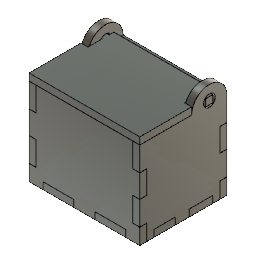
Music Box v1 (Autodesk Fusion 360 design; units mm, degrees)
Autodesk Fusion 360 part; units mm, degrees
sketch "Sketch1" plane through (0, 0, 0) normal (0, 0, 1) x (1, 0, 0)
  line L0 (0, 0) -> (47, 0)
  line L1 (47, 0) -> (47, 37)
  line L2 (47, 37) -> (0, 37)
  line L3 (0, 37) -> (0, 0)
  dimension "d1" = 47
  dimension "d2" = 37
  constraint horizontal L0
  constraint vertical L1
  constraint horizontal L2
  constraint vertical L3
  constraint coincident L0.start L3.end
  measures "d1" distance of L0.start L0.end
  measures "d2" distance of L0.start L2.end
sketch "Sketch2" plane through (0, 0, 0) normal (0, 0, 1) x (1, 0, 0)
  line L0 (0, 0) -> (3, 0)
  line L1 (3, 0) -> (3, 3)
  line L2 (3, 3) -> (0, 3)
  line L3 (0, 3) -> (0, 0)
  line L4 (25, 0) -> (25, 3)
  line L5 (22, 0) -> (25, 0)
  line L6 (25, 3) -> (22, 3)
  line L7 (22, 3) -> (22, 0)
  line L8 (47, 0) -> (47, 3)
  line L9 (44, 0) -> (47, 0)
  line L10 (47, 3) -> (44, 3)
  line L11 (44, 3) -> (44, 0)
  line L12 (25, 0) -> (28, 0)
  line L13 (28, 0) -> (28, 3)
  line L14 (25, 3) -> (25, 0)
  line L15 (28, 3) -> (25, 3)
  line L16 (22, 3) -> (19, 3)
  line L17 (22, 3) -> (22, 0)
  line L18 (19, 0) -> (22, 0)
  line L19 (19, 3) -> (19, 0)
  line L20 (6, 3) -> (3, 3)
  line L21 (6, 0) -> (6, 3)
  line L22 (3, 0) -> (6, 0)
  line L23 (3, 3) -> (3, 0)
  line L24 (41, 3) -> (41, 0)
  line L25 (44, 3) -> (41, 3)
  line L26 (41, 0) -> (44, 0)
  line L27 (44, 0) -> (44, 3)
  line L28 (19, 37) -> (19, 34)
  line L29 (28, 34) -> (28, 37)
  line L30 (25, 34) -> (28, 34)
  line L31 (22, 34) -> (25, 34)
  line L32 (28, 37) -> (25, 37)
  line L33 (25, 37) -> (22, 37)
  line L34 (22, 37) -> (19, 37)
  line L35 (6, 37) -> (3, 37)
  line L36 (6, 34) -> (6, 37)
  line L37 (3, 34) -> (6, 34)
  line L38 (0, 34) -> (3, 34)
  line L39 (0, 37) -> (0, 34)
  line L40 (3, 37) -> (0, 37)
  line L41 (41, 37) -> (41, 34)
  line L42 (44, 37) -> (41, 37)
  line L43 (47, 37) -> (44, 37)
  line L44 (41, 34) -> (44, 34)
  line L45 (44, 34) -> (47, 34)
  line L46 (47, 34) -> (47, 37)
  line L47 (19, 34) -> (22, 34)
  line L48 (47, 0) -> (47, 3)
  line L49 (47, 3) -> (44, 3)
  line L50 (44, 3) -> (44, 0)
  line L51 (44, 0) -> (47, 0)
  line L52 (3, 31) -> (3, 34)
  line L53 (3, 34) -> (0, 34)
  line L54 (0, 34) -> (0, 31)
  line L55 (0, 31) -> (3, 31)
  line L56 (47, 31) -> (47, 34)
  line L57 (47, 34) -> (44, 34)
  line L58 (44, 34) -> (44, 31)
  line L59 (44, 31) -> (47, 31)
  line L60 (3, 3) -> (3, 6)
  line L61 (0, 3) -> (3, 3)
  line L62 (0, 6) -> (0, 3)
  line L63 (3, 6) -> (0, 6)
  line L64 (44, 6) -> (44, 3)
  line L65 (44, 3) -> (47, 3)
  line L66 (47, 6) -> (44, 6)
  line L67 (47, 3) -> (47, 6)
  line L68 (44, 15) -> (47, 15)
  line L69 (47, 15) -> (47, 18)
  line L70 (47, 18) -> (47, 21)
  line L71 (47, 21) -> (44, 21)
  line L72 (44, 21) -> (44, 18)
  line L73 (44, 15) -> (44, 18)
  line L74 (3, 18) -> (3, 21)
  line L75 (3, 21) -> (0, 21)
  line L76 (0, 21) -> (0, 18)
  line L77 (0, 18) -> (0, 15)
  line L78 (0, 15) -> (3, 15)
  line L79 (3, 18) -> (3, 15)
  point P0 (0, 6)
  dimension "d9" = 3
  dimension "d10" = 3
  dimension "d13" = 44
  dimension "d14" = 0
  dimension "d17" = 3
  dimension "d18" = 0
  dimension "d21" = -3
  dimension "d22" = 0
  dimension "d25" = 3
  dimension "d26" = 0
  dimension "d29" = -3
  dimension "d30" = 0
  dimension "d33" = 0
  dimension "d34" = 34
  dimension "d37" = 44
  dimension "d38" = 31
  dimension "d41" = 0
  dimension "d42" = -28
  dimension "d45" = 0
  dimension "d46" = 15
  constraint horizontal L0
  constraint vertical L1
  constraint horizontal L2
  constraint vertical L3
  constraint coincident L0.start L3.end
  measures "d9" distance of L0.start L0.end
  measures "d10" distance of L0.start L2.end
extrude "Extrude1" add sketch "Sketch1" along normal blind 3 makes body 1
extrude "Extrude2" cut sketch "Sketch2" along normal blind 3 bodies 1
sketch "Sketch3" plane through (0, 0, 0) normal (0, 0, 1) x (1, 0, 0)
  line L0 (0, 0) -> (47, 0)
  line L1 (47, 0) -> (47, 3)
  line L2 (47, 3) -> (0, 3)
  line L3 (0, 3) -> (0, 0)
  dimension "d51" = 47
  dimension "d52" = 3
  constraint horizontal L0
  constraint vertical L1
  constraint horizontal L2
  constraint vertical L3
  constraint coincident L0.start L3.end
  measures "d51" distance of L0.start L0.end
  measures "d52" distance of L0.start L2.end
extrude "Extrude1'" add sketch "Sketch3" along normal blind 37 separate body makes body 2 in component "Component"
sketch "Sketch4" plane through (0, 0, 0) normal (0, -1, 0) x (1, 0, 0)
  line L0 (0, 0) -> (47, 0)
  line L1 (47, 0) -> (47, 37)
  line L2 (47, 37) -> (0, 37)
  line L3 (0, 37) -> (0, 0)
  line L4 (0, 37) -> (3, 37)
  line L5 (3, 37) -> (3, 26.7867)
  line L6 (3, 26.7867) -> (0, 26.7867)
  line L7 (0, 26.7867) -> (0, 37)
  line L8 (44, 37) -> (47, 37)
  line L9 (47, 37) -> (47, 26.7867)
  line L10 (44, 26.7867) -> (44, 37)
  line L11 (47, 26.7867) -> (44, 26.7867)
  line L12 (0, 17) -> (3, 17)
  line L13 (3, 17) -> (3, 6.7867)
  line L14 (0, 6.7867) -> (0, 17)
  line L15 (3, 6.7867) -> (0, 6.7867)
  line L16 (44, 17) -> (47, 17)
  line L17 (47, 17) -> (47, 6.7867)
  line L18 (44, 6.7867) -> (44, 17)
  line L19 (47, 6.7867) -> (44, 6.7867)
  line L20 (19, 0) -> (6, 0)
  line L21 (6, 0) -> (6, 3)
  line L22 (6, 3) -> (19, 3)
  line L23 (19, 3) -> (19, 0)
  line L24 (41, 3) -> (41, 0)
  line L25 (41, 0) -> (28, 0)
  line L26 (28, 3) -> (41, 3)
  line L27 (28, 0) -> (28, 3)
  dimension "d55" = 3
  dimension "d56" = 10.2133
  dimension "d59" = 44
  dimension "d60" = -20
  dimension "d61" = 13
  dimension "d62" = 3
  dimension "d65" = 22
  dimension "d66" = 0
  constraint horizontal L4
  constraint vertical L5
  constraint horizontal L6
  constraint vertical L7
  constraint coincident L2.end L3.start
  constraint horizontal L20
  constraint vertical L21
  constraint horizontal L22
  constraint vertical L23
  constraint coincident L0 L20.start
  measures "d55" distance of L2.end L4.end
  measures "d56" distance of L2.end L6.end
  measures "d61" distance of L20.start L20.end
  measures "d62" distance of L20.start L22.end
extrude "Extrude2'" cut sketch "Sketch4" against normal blind 3 contours L0 L20 L21 L22 L23 | L3 L12 L13 L14 L15 | L0 L24 L25 L26 L27 | L2 L3 L4 L5 L6 L7 | L1 L16 L17 L18 L19 | L1 L2 L8 L9 L10 L11 bodies 2 in component "Component"
sketch "Sketch5" plane through (0, 0, 0) normal (-1, 0, 0) x (0, -1, 0)
  line L0 (0, 26.7867) -> (-3, 26.7867)
  line L1 (-3, 26.7867) -> (-3, 17)
  line L2 (-3, 17) -> (0, 17)
  line L3 (0, 17) -> (0, 26.7867)
  line L4 (0, 0) -> (-37, 0)
  line L5 (-37, 0) -> (-37, 37)
  line L6 (-37, 37) -> (0, 37)
  line L7 (0, 37) -> (0, 0)
  line L8 (0, 6.816) -> (-3, 6.816)
  line L9 (-3, 6.816) -> (-3, 0)
  line L10 (-3, 0) -> (0, 0)
  line L11 (0, 0) -> (0, 6.816)
  dimension "d69" = 37
  dimension "d70" = 37
  constraint horizontal L4
  constraint vertical L5
  constraint horizontal L6
  constraint vertical L7
  constraint coincident L4.start L7.end
  constraint horizontal L8
  constraint vertical L9
  constraint horizontal L10
  constraint vertical L11
  constraint coincident L4 L9.end
  constraint coincident L7 L8.start
  measures "d69" distance of L4.start L4.end
  measures "d70" distance of L4.start L6.end
sketch "Sketch6" plane through (0, 0, 0) normal (-1, 0, 0) x (0, -1, 0)
  line L0 (-3, 6.816) -> (0, 6.816)
  line L1 (0, 6.816) -> (0, 17)
  line L2 (0, 17) -> (-3, 17)
  line L3 (-3, 17) -> (-3, 26.7867)
  line L4 (-3, 26.7867) -> (0, 26.7867)
  line L5 (0, 26.7867) -> (0, 37)
  line L6 (0, 37) -> (-37, 37)
  line L7 (-37, 37) -> (-37, 0)
  line L8 (-37, 0) -> (-3, 0)
  line L9 (-3, 0) -> (-3, 6.816)
  line L10 (-37, 26.7867) -> (-34, 26.7867)
  line L11 (-37, 17) -> (-37, 26.7867)
  line L12 (-34, 17) -> (-37, 17)
  line L13 (-37, 6.816) -> (-34, 6.816)
  line L14 (-37, 0) -> (-37, 6.816)
  spline S0 degree 5 poles (-34, 26.7867) (-34, 26.3953) (-34, 25.6123) (-34, 24.4379) (-34, 22.872) (-34, 20.9147) (-34, 19.3488) (-34, 18.1744) (-34, 17.3915) (-34, 17) knots 0 0 0 0 0 0 0.2 0.4 0.6 0.8 1 1 1 1 1 1
  spline S1 degree 5 poles (-34, 6.816) (-34, 6.5433) (-34, 5.9981) (-34, 5.1801) (-34, 4.0896) (-34, 2.7264) (-34, 1.6358) (-34, 0.8179) (-34, 0.2726) (-34, 0) knots 0 0 0 0 0 0 0.2 0.4 0.6 0.8 1 1 1 1 1 1
  spline S2 degree 5 poles (-37, 0) (-36.88, 0) (-36.64, 0) (-36.28, 0) (-35.8, 0) (-35.2, 0) (-34.72, 0) (-34.36, 0) (-34.12, 0) (-34, 0) knots 0 0 0 0 0 0 0.2 0.4 0.6 0.8 1 1 1 1 1 1
  line L15 (-31, 3) -> (-26, 3)
  line L16 (-26, 3) -> (-26, 0)
  line L17 (-26, 0) -> (-31, 0)
  line L18 (-31, 0) -> (-31, 3)
  line L19 (-26, 3) -> (-21, 3)
  line L20 (-26, 0) -> (-26, 3)
  line L21 (-21, 3) -> (-21, 0)
  line L22 (-21, 0) -> (-26, 0)
  line L23 (-15, 0) -> (-12, 0)
  line L24 (-12, 0) -> (-12, 3)
  line L25 (-12, 3) -> (-15, 3)
  line L26 (-15, 3) -> (-15, 0)
  line L27 (-9, 3) -> (-12, 3)
  line L28 (-12, 3) -> (-12, 0)
  line L29 (-12, 0) -> (-9, 0)
  line L30 (-9, 0) -> (-9, 3)
  line L31 (-6, 3) -> (-9, 3)
  line L32 (-9, 3) -> (-9, 0)
  line L33 (-9, 0) -> (-6, 0)
  line L34 (-6, 0) -> (-6, 3)
  dimension "d75" = -34
  dimension "d76" = 0
  dimension "d77" = 5
  dimension "d78" = 3
  dimension "d81" = 5
  dimension "d82" = 0
  dimension "d83" = 3
  dimension "d84" = 3
  dimension "d87" = 6
  dimension "d88" = 0
  constraint coincident L8 S1.end
  constraint coincident L7.end L8.start
  constraint horizontal L15
  constraint vertical L16
  constraint horizontal L17
  constraint vertical L18
  constraint horizontal L23
  constraint vertical L24
  constraint horizontal L25
  constraint vertical L26
  measures "d77" distance of L15.start L15.end
  measures "d78" distance of L15.start L17.end
  measures "d83" distance of L23.start L23.end
  measures "d84" distance of L23.start L25.end
extrude "Extrude1''" add sketch "Sketch6" against normal blind 3 separate body contours L0 L1 L2 L3 L4 L5 L6 L7 L8 L9 L10 L12 L13 S0 S1 L15 L18 L19 L21 L25 L26 L27 L31 L34 makes body 3 in component "Component'"
extrude "Extrude1'''" add 1 faces at (22, 0, 18.8578) along direction (0, -1, 0) blind -37 and the other way blind 34 separate body on bodies 2 makes body 4 in component "Component''"
extrude "Extrude1''''" add 1 faces at (3, 19.3333, 12.3333) along direction (1, 0, 0) blind 41 and the other way blind -44 separate body on bodies 3 makes body 5 in component "Component'''"
extrude "Extrude3" cut 1 faces at (16.6667, 2, 37) along direction (0, 0, -1) blind 3 on bodies 2 bodies 2 in component "Component"
sketch "Sketch7" plane through (47, 0, 0) normal (1, 0, 0) x (0, 1, 0)
  line L0 (3, 6.816) -> (3, 0)
  line L1 (3, 0) -> (6, 0)
  line L2 (6, 0) -> (6, 3)
  line L3 (6, 3) -> (15, 3)
  line L4 (15, 3) -> (15, 0)
  line L5 (15, 0) -> (21, 0)
  line L6 (21, 0) -> (21, 3)
  line L7 (21, 3) -> (31, 3)
  line L8 (31, 3) -> (31, 0)
  line L9 (31, 0) -> (34, 0)
  line L10 (34, 0) -> (34, 6.816)
  line L11 (34, 6.816) -> (37, 6.816)
  line L12 (37, 6.816) -> (37, 17)
  line L13 (37, 17) -> (34, 17)
  line L14 (34, 17) -> (34, 26.7867)
  line L15 (34, 26.7867) -> (37, 26.7867)
  line L16 (37, 26.7867) -> (37, 37)
  line L17 (37, 37) -> (0, 37)
  line L18 (0, 37) -> (0, 26.7867)
  line L19 (0, 26.7867) -> (3, 26.7867)
  line L20 (3, 26.7867) -> (3, 17)
  line L21 (3, 17) -> (0, 17)
  line L22 (0, 17) -> (0, 6.816)
  line L23 (0, 6.816) -> (3, 6.816)
  circle A0 centre (29.5075, 37) radius 7.5
  dimension "d101" = 15
  constraint coincident L17 A0.centre
  measures "d101" diameter of A0
extrude "Extrude2''" add sketch "Sketch7" against normal blind 3 contours L16 L17 A0 picked at (27.0329, 37.3726) bodies 5 in component "Component'''"
sketch "Sketch8" plane through (0, 0, 0) normal (-1, 0, 0) x (0, -1, 0)
  line L0 (-3, 0) -> (-3, 6.816)
  line L1 (-3, 6.816) -> (0, 6.816)
  line L2 (0, 6.816) -> (0, 17)
  line L3 (0, 17) -> (-3, 17)
  line L4 (-3, 17) -> (-3, 26.7867)
  line L5 (-3, 26.7867) -> (0, 26.7867)
  line L6 (0, 26.7867) -> (0, 37)
  line L7 (0, 37) -> (-37, 37)
  line L8 (-37, 37) -> (-37, 26.7867)
  line L9 (-37, 26.7867) -> (-34, 26.7867)
  line L10 (-34, 26.7867) -> (-34, 17)
  line L11 (-34, 17) -> (-37, 17)
  line L12 (-37, 17) -> (-37, 6.816)
  line L13 (-37, 6.816) -> (-34, 6.816)
  line L14 (-34, 6.816) -> (-34, 0)
  line L15 (-34, 0) -> (-31, 0)
  line L16 (-31, 0) -> (-31, 3)
  line L17 (-31, 3) -> (-21, 3)
  line L18 (-21, 3) -> (-21, 0)
  line L19 (-21, 0) -> (-15, 0)
  line L20 (-15, 0) -> (-15, 3)
  line L21 (-15, 3) -> (-6, 3)
  line L22 (-6, 3) -> (-6, 0)
  line L23 (-6, 0) -> (-3, 0)
  circle A0 centre (-29.4944, 37) radius 7.5
  dimension "d104" = 15
  constraint coincident L7 A0.centre
  measures "d104" diameter of A0
extrude "Extrude2'''" add sketch "Sketch8" against normal blind 3 contours L7 A0 picked at (-30.0507, 39.4373) bodies 3 in component "Component'"
extrude "Extrude4" add 1 faces at (16.6667, 2, 34) along direction (0, 0, 1) blind 3 on bodies 2 bodies 2 in component "Component"
sketch "Sketch9" plane through (0, 0, 3) normal (0, 0, 1) x (-1, 0, 0)
  line L0 (-41, 0) -> (-41, -3)
  line L1 (-41, -3) -> (-44, -3)
  line L2 (-44, -3) -> (-44, -6)
  line L3 (-44, -6) -> (-47, -6)
  line L4 (-47, -6) -> (-47, -15)
  line L5 (-47, -15) -> (-44, -15)
  line L6 (-44, -15) -> (-44, -21)
  line L7 (-44, -21) -> (-47, -21)
  line L8 (-47, -21) -> (-47, -31)
  line L9 (-47, -31) -> (-44, -31)
  line L10 (-44, -31) -> (-44, -34)
  line L11 (-44, -34) -> (-41, -34)
  line L12 (-41, -34) -> (-41, -37)
  line L13 (-41, -37) -> (-28, -37)
  line L14 (-28, -37) -> (-28, -34)
  line L15 (-28, -34) -> (-19, -34)
  line L16 (-19, -34) -> (-19, -37)
  line L17 (-19, -37) -> (-6, -37)
  line L18 (-6, -37) -> (-6, -34)
  line L19 (-6, -34) -> (-3, -34)
  line L20 (-3, -34) -> (-3, -31)
  line L21 (-3, -31) -> (0, -31)
  line L22 (0, -31) -> (0, -21)
  line L23 (0, -21) -> (-3, -21)
  line L24 (-3, -21) -> (-3, -15)
  line L25 (-3, -15) -> (0, -15)
  line L26 (0, -15) -> (0, -6)
  line L27 (0, -6) -> (-3, -6)
  line L28 (-3, -6) -> (-3, -3)
  line L29 (-3, -3) -> (-6, -3)
  line L30 (-6, -3) -> (-6, 0)
  line L31 (-6, 0) -> (-19, 0)
  line L32 (-19, 0) -> (-19, -3)
  line L33 (-19, -3) -> (-28, -3)
  line L34 (-28, -3) -> (-28, 0)
  line L35 (-28, 0) -> (-41, 0)
  line L36 (0, 0) -> (-47, 0)
  line L37 (-47, 0) -> (-47, -37)
  line L38 (-47, -37) -> (0, -37)
  line L39 (0, -37) -> (0, 0)
  dimension "d109" = 47
  dimension "d110" = 37
  constraint horizontal L36
  constraint vertical L37
  constraint horizontal L38
  constraint vertical L39
  constraint coincident L36.start L39.end
  measures "d109" distance of L36.start L36.end
  measures "d110" distance of L36.start L38.end
extrude "Extrude1'''''" add sketch "Sketch9" along normal blind 37 and the other way blind -34 separate body makes body 6 in component "Component''''"
sketch "Sketch10" plane through (0, 0, 40) normal (0, 0, 1) x (-1, 0, 0)
  line L0 (0, -37) -> (0, 0)
  line L1 (0, 0) -> (-47, 0)
  line L2 (-47, 0) -> (-47, -37)
  line L3 (-47, -37) -> (0, -37)
  line L4 (0, -37) -> (-3, -37)
  line L5 (-3, -37) -> (-3, -22)
  line L6 (-3, -22) -> (0, -22)
  line L7 (0, -22) -> (0, -37)
  line L8 (-44, -37) -> (-47, -37)
  line L9 (-47, -37) -> (-47, -22)
  line L10 (-44, -22) -> (-44, -37)
  line L11 (-47, -22) -> (-44, -22)
  dimension "d117" = -44
  dimension "d118" = 0
  constraint horizontal L4
  constraint vertical L5
  constraint horizontal L6
  constraint vertical L7
  constraint coincident L0.start L3.end
extrude "Extrude2''''" cut sketch "Sketch10" against normal blind 3 contours L0 L3 L4 L5 L6 L7 | L2 L3 L8 L9 L10 L11 bodies 6 in component "Component''''"
sketch "Sketch11" plane through (0, 0, 40) normal (0, 0, 1) x (-1, 0, 0)
  line L0 (-3, -22) -> (0, -22)
  line L1 (0, -22) -> (0, 0)
  line L2 (0, 0) -> (-47, 0)
  line L3 (-47, 0) -> (-47, -22)
  line L4 (-47, -22) -> (-44, -22)
  line L5 (-44, -22) -> (-44, -37)
  line L6 (-44, -37) -> (-3, -37)
  line L7 (-3, -37) -> (-3, -22)
  line L8 (-3, -37) -> (-44, -37)
  line L9 (-44, -37) -> (-44, -34)
  line L10 (-44, -34) -> (-3, -34)
  line L11 (-3, -34) -> (-3, -37)
  dimension "d121" = 3
  constraint horizontal L8
  constraint vertical L9
  constraint horizontal L10
  constraint vertical L11
  constraint coincident L6.end L7.start
  measures "d121" distance of L6.end L10.end
extrude "Extrude3'" cut sketch "Sketch11" against normal blind 3 contours L5 L6 L7 L8 L9 L10 L11 bodies 6 in component "Component''''"
sketch "Sketch12" plane through (0, 0, 40) normal (0, 0, 1) x (-1, 0, 0)
  line L0 (-44, -34) -> (-3, -34)
  line L1 (-3, -34) -> (-3, -22)
  line L2 (-3, -22) -> (0, -22)
  line L3 (0, -22) -> (0, 0)
  line L4 (0, 0) -> (-47, 0)
  line L5 (-47, 0) -> (-47, -22)
  line L6 (-47, -22) -> (-44, -22)
  line L7 (-44, -22) -> (-44, -34)
hole "Hole1" at (47, 29.5396, 38.575) direction (-1, 0, 0) diameter 5 depth 49 tip angle 118 bodies 3 in component "Component'"
hole "Hole1'" at (47, 29.5396, 38.575) direction (-1, 0, 0) diameter 5 depth 49 tip angle 118 bodies 5 in component "Component'''"
sketch "Sketch13" plane through (0, 0, 40) normal (0, 0, 1) x (1, 0, 0)
  line L0 (3, 31) -> (0, 31)
  line L1 (0, 31) -> (0, 28)
  line L2 (0, 28) -> (3, 28)
  line L3 (3, 28) -> (3, 31)
  constraint horizontal L0
  constraint vertical L1
  constraint horizontal L2
  constraint vertical L3
extrude "Extrude4'" add sketch "Sketch13" against normal blind 3 bodies 6 in component "Component''''"
sketch "Sketch14" plane through (0, 0, 3) normal (0, 0, 1) x (-1, 0, 0)
  line L0 (-41, 0) -> (-41, -3)
  line L1 (-41, -3) -> (-44, -3)
  line L2 (-44, -3) -> (-44, -6)
  line L3 (-44, -6) -> (-47, -6)
  line L4 (-47, -6) -> (-47, -15)
  line L5 (-47, -15) -> (-44, -15)
  line L6 (-44, -15) -> (-44, -21)
  line L7 (-44, -21) -> (-47, -21)
  line L8 (-47, -21) -> (-47, -31)
  line L9 (-47, -31) -> (-44, -31)
  line L10 (-44, -31) -> (-44, -34)
  line L11 (-44, -34) -> (-41, -34)
  line L12 (-41, -34) -> (-41, -37)
  line L13 (-41, -37) -> (-28, -37)
  line L14 (-28, -37) -> (-28, -34)
  line L15 (-28, -34) -> (-19, -34)
  line L16 (-19, -34) -> (-19, -37)
  line L17 (-19, -37) -> (-6, -37)
  line L18 (-6, -37) -> (-6, -34)
  line L19 (-6, -34) -> (-3, -34)
  line L20 (-3, -34) -> (-3, -31)
  line L21 (-3, -31) -> (0, -31)
  line L22 (0, -31) -> (0, -21)
  line L23 (0, -21) -> (-3, -21)
  line L24 (-3, -21) -> (-3, -15)
  line L25 (-3, -15) -> (0, -15)
  line L26 (0, -15) -> (0, -6)
  line L27 (0, -6) -> (-3, -6)
  line L28 (-3, -6) -> (-3, -3)
  line L29 (-3, -3) -> (-6, -3)
  line L30 (-6, -3) -> (-6, 0)
  line L31 (-6, 0) -> (-19, 0)
  line L32 (-19, 0) -> (-19, -3)
  line L33 (-19, -3) -> (-28, -3)
  line L34 (-28, -3) -> (-28, 0)
  line L35 (-28, 0) -> (-41, 0)
sketch "Sketch15" plane through (0, 0, 0) normal (0, 1, 0) x (1, 0, 0)
  line L0 (47, -40) -> (44, -40)
  line L1 (44, -40) -> (44, -37)
  line L2 (44, -37) -> (47, -37)
  line L3 (47, -37) -> (47, -40)
  dimension "d132" = 3
  dimension "d133" = 3
  constraint horizontal L0
  constraint vertical L1
  constraint horizontal L2
  constraint vertical L3
  measures "d132" distance of L0.start L0.end
  measures "d133" distance of L0.start L2.end
extrude "Extrude5" add sketch "Sketch15" along normal blind 31 and the other way blind -28 bodies 6 in component "Component''''"
sketch "Sketch16" plane through (0, 0, 40) normal (0, 0, 1) x (1, 0, 0)
  line L0 (44, 34) -> (3, 34)
  line L1 (3, 34) -> (3, 33)
  line L2 (3, 33) -> (44, 33)
  line L3 (44, 33) -> (44, 34)
  constraint horizontal L0
  constraint vertical L1
  constraint horizontal L2
  constraint vertical L3
extrude "Extrude6" cut sketch "Sketch16" against normal blind 3 bodies 6 in component "Component''''"
component "Component" placed x (1, 0, 0) y (0, 1, 0) z (0, 0, 1) at (0, 0, 0)
component "Component'" placed x (1, 0, 0) y (0, 1, 0) z (0, 0, 1) at (0, 0, 0)
component "Component''" placed x (1, 0, 0) y (0, 1, 0) z (0, 0, 1) at (0, 0, 0)
component "Component'''" placed x (1, 0, 0) y (0, 1, 0) z (0, 0, 1) at (0, 0, 0)
component "Component''''" placed x (1, 0, 0) y (0, 1, 0) z (0, 0, 1) at (0, 0, 0)
equation "boxside = 37 mm" comment "box side short"
equation "boxsidelong = 47 mm" comment "box side long"
equation "boxthickness = 3 mm" comment "box thickness"
equation "boxholeheight = 5 mm" comment "box hole"
equation "boxcorner = 15 mm" comment "circular box corner (top)"
equation "boxhole = 5 mm" comment "box hole for cover"
equation "d9 = boxthickness"
equation "d10 = boxthickness"
equation "d47 = boxthickness"
equation "d51 = boxsidelong"
equation "d52 = boxthickness"
equation "d53 = boxside"
equation "d55 = boxthickness"
equation "d62 = boxthickness"
equation "d69 = boxside"
equation "d70 = boxside"
equation "d77 = boxhole"
equation "d78 = boxthickness"
equation "d83 = boxthickness"
equation "d84 = boxthickness"
equation "d91 = -boxside"
equation "d99 = -boxthickness"
equation "d101 = boxcorner"
equation "d104 = boxcorner"
equation "d109 = boxsidelong"
equation "d110 = boxside"
equation "d119 = -boxthickness"
equation "d121 = boxthickness"
